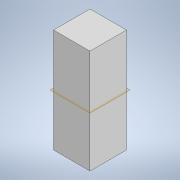
# Autodesk Inventor part: latticeStandIn
Saved by Autodesk Inventor 2020 (Build 240168000, 168)
## iProperties
Created: 2022-09-27
Part Number: latticeStandIn
Material: Generic
Document SubType Name: Modeling
Designer: iss
Density: 1 g/cm^3
Appearance: Default
Author: iss
Autodesk Inventor part; units mm, degrees
ref_plane "YZ Plane" through (0, 0, 0) normal (1, 0, 0) x (0, 1, 0)
ref_plane "XZ Plane" through (0, 0, 0) normal (0, 1, 0) x (-1, 0, 0)
ref_plane "XY Plane" through (0, 0, 0) normal (0, 0, 1) x (1, 0, 0)
sketch "Sketch1" plane through (0, 0, 0) normal (0, 1, 0) x (-1, 0, 0)
  line L0 (6.5, 0) -> (0, 0)
  line L1 (0, 0) -> (0, -6.5)
  line L2 (6.5, 0) -> (6.5, -6.5)
  line L3 (6.5, -6.5) -> (0, -6.5)
  dimension "d0" = 6.5
  dimension "d1" = 6.5
  constraints: 8 end point, 3 perpendicular, 1 horizontal
  measures "d0" distance of L0.end L1.end
  measures "d1" distance of L0.start L0.end
extrude "Extrusion1" add sketch "Sketch1" along normal blind 18.5
ref_plane "Work Plane1" through (0, 9.25, 0) normal (0, 1, 0) x (1, 0, 0)
body "Solid1"
